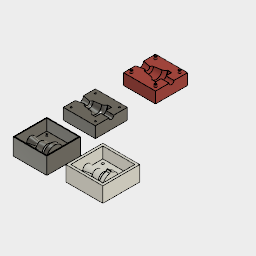
knobv8 (Autodesk Fusion 360 design; units mm, degrees)
Autodesk Fusion 360 part; units mm, degrees
sketch "Sketch1" plane through (0, 0, 0) normal (0, 0, 1) x (1, 0, 0)
  circle A0 centre (0, 0) radius 10
  line L0 (0, 13) -> (-1.5, 9.5)
  line L1 (-1.5, 9.5) -> (1.5, 9.5)
  line L2 (1.5, 9.5) -> (0, 13)
extrude "Extrude1" add sketch "Sketch1" along normal blind 5 makes body 1
sketch "Sketch2" plane through (0, 0, 5) normal (0, 0, 1) x (-1, 0, 0)
  arc A0 (1.3234, -9.912) -> (-1.3234, -9.912) centre (0, 0) ccw
  line L0 (-1.3234, -9.912) -> (0, -13)
  line L1 (0, -13) -> (1.3234, -9.912)
  circle A1 centre (0, 0) radius 7.5
  dimension "d3" = 15
  measures "d3" diameter of A1
ref_plane "WorkPlane1" through (0, 0, 20) normal (0, 0, 1) x (-1, 0, 0)
sketch "Sketch3" plane through (0, 0, 20) normal (0, 0, 1) x (1, 0, 0)
  circle A0 centre (0, 0) radius 5
loft "Loft1" add profiles "Sketch3", "Sketch2" section 1 section 2 contours A1 bodies 1
fillet "Fillet1" radius 0.5 3 edges at (0, -10, 5) (-0.6617, 11.456, 5) (0.6617, 11.456, 5) on bodies 1
fillet "Fillet2" radius 2.5 1 edges at (-4.6616, 1.8081, 20) on bodies 1
fillet "Fillet3" radius 5.5 1 edges at (6.9925, -2.7121, 5) on bodies 1
fillet "Fillet4" radius 0.5 2 edges at (0, 13, 2.25) (0, 12.6282, 4.8536) on bodies 1
sketch "Sketch5" plane through (0, 0, 0) normal (0, 0, -1) x (1, 0, 0)
  arc A0 (-0.4596, -11.9277) -> (0.4596, -11.9277) centre (0, -11.7307) ccw
  line L0 (0.4596, -11.9277) -> (1.3234, -9.912)
  arc A1 (1.3234, -9.912) -> (-1.3234, -9.912) centre (0, 0) ccw
  line L1 (-1.3234, -9.912) -> (-0.4596, -11.9277)
  line L2 (-15, 0) -> (15.3298, 0)
  line L3 (15.3298, 0) -> (15.3298, 10)
  line L4 (15.3298, 10) -> (-15, 10)
  line L5 (-15, 10) -> (-15, 0)
copy_body "CopyPasteBodies1" bodies 1 makes body 2
move_body "Move1" bodies 2 to x (1, 0, 0) y (0, 1, 0) z (0, 0, 1) at (-44, 0, 0)
extrude "Extrude3" cut sketch "Sketch5" along normal blind -22 and the other way blind -3 contours A1 L2 L4 L5 | A1 L2 | A1 L2 L3 L4 bodies 1
sketch "Sketch6" plane through (0, 0, 0) normal (0, 0, -1) x (1, 0, 0)
  arc A0 (-44.4596, -11.9277) -> (-43.5404, -11.9277) centre (-44, -11.7307) ccw
  line L0 (-43.5404, -11.9277) -> (-42.6766, -9.912)
  arc A1 (-42.6766, -9.912) -> (-45.3234, -9.912) centre (-44, 0) ccw
  line L1 (-45.3234, -9.912) -> (-44.4596, -11.9277)
  line L2 (-60, 0) -> (-30, 0)
  line L3 (-30, 0) -> (-30, -13)
  line L4 (-30, -13) -> (-60, -13)
  line L5 (-60, -13) -> (-60, 0)
extrude "Extrude4" cut sketch "Sketch6" along normal blind -22 and the other way blind -1 contours A0 L0 A1 L1 L2 | A0 L0 A1 L1 L2 L3 L4 L5 bodies 2
move_body "Move2" bodies 2 to x (1, 0, 0) y (0, 0, -1) z (0, 1, 0) at (0, -5, -5)
sketch "Sketch7" plane through (0, 0, 0) normal (0, 0, 1) x (1, 0, 0)
  line L0 (-65, 25) -> (-25, 25)
  line L1 (-25, 25) -> (-25, -15)
  line L2 (-25, -15) -> (-65, -15)
  line L3 (-65, -15) -> (-65, 25)
move_body "Align1" bodies 2 to x (0, 1, 0) y (-1, 0, 0) z (0, 0, 1) at (-70, 39, 5)
extrude "Extrude5" add sketch "Sketch7" against normal blind 5 separate body makes body 3
move_body "Align2" bodies 2 to x (1, 0, 0) y (0, 1, 0) z (0, 0, 1) at (30, 10, 0)
sketch "Sketch8" plane through (-65, 0, 0) normal (-1, 0, 0) x (0, -1, 0)
  line L0 (15, 0) -> (-25, 0)
  line L1 (-25, 0) -> (-25, -5)
  line L2 (-25, -5) -> (15, -5)
  line L3 (15, -5) -> (15, 0)
  circle A0 centre (-5, 0) radius 5
loft "Loft2" add profiles "Sketch8" section 1 contours L0 A0 picked at (-5.7088, 3.1054) section 2 face at (-55, 6.2273, 1.168) on bodies 2 bodies 2 3
move_body "Move3" bodies 1 to x (1, 0, 0) y (0, 1, 0) z (0, 0, 1) at (-43.1702, -52.4938, 0)
sketch "Sketch9" plane through (-35, 0, 0) normal (1, 0, 0) x (0, 1, 0)
  line L0 (-5, 0) -> (15, 0)
  arc A0 (15, 0) -> (-5, 0) centre (5, 0) ccw
  circle A1 centre (5, 0) radius 3
  dimension "d24" = 6
  measures "d24" diameter of A1
extrude "Extrude6" add sketch "Sketch9" along normal blind 10 contours L0 A1 picked at (5.9556, 0.2948) bodies 2
sketch "Sketch10" plane through (0, 0, -5) normal (0, 0, -1) x (1, 0, 0)
  line L0 (-25, 15) -> (-65, 15)
  line L1 (-65, 15) -> (-65, -25)
  line L2 (-65, -25) -> (-25, -25)
  line L3 (-25, -25) -> (-25, 15)
  line L4 (-75, 25) -> (-15, 25)
  line L5 (-15, 25) -> (-15, -35)
  line L6 (-15, -35) -> (-75, -35)
  line L7 (-75, -35) -> (-75, 25)
  line L8 (-78, -38) -> (-78, 28)
  line L9 (-78, 28) -> (-12, 28)
  line L10 (-12, 28) -> (-12, -38)
  line L11 (-12, -38) -> (-78, -38)
  dimension "d27" = 3
extrude "Extrude7" add sketch "Sketch10" against normal blind 15 contours L4 L5 L6 L7 bodies 2
sketch "Sketch11" plane through (0, 0, 0) normal (0, 0, 1) x (-1, 0, 0)
  line L0 (35, -8) -> (25, -8)
  line L1 (25, -8) -> (25, -25)
  line L2 (25, -25) -> (65, -25)
  line L3 (65, -25) -> (65, -10)
  line L4 (65, -10) -> (55, -7.8822)
  arc A0 (52.911, -10.3482) -> (55, -7.8822) centre (52.5, -7.8822) ccw
  line L5 (52.911, -10.3482) -> (43.9169, -11.8472)
  arc A1 (43.9169, -11.8472) -> (39.9434, -14.731) centre (44.8211, -17.2723) ccw
  arc A2 (39.5, -15) -> (39.9434, -14.731) centre (39.5, -14.5) ccw
  line L6 (39.5, -15) -> (35, -15)
  line L7 (35, -15) -> (35, -8)
  circle A3 centre (60, -20) radius 1
  circle A4 centre (30, -20) radius 1
  dimension "d39" = 2
  dimension "d40" = 2
  measures "d39" diameter of A4
  measures "d40" diameter of A3
sketch "Sketch12" plane through (0, 0, 0) normal (0, 0, 1) x (-1, 0, 0)
  line L0 (25, -2) -> (35, -2)
  line L1 (35, -2) -> (35, 5)
  line L2 (35, 5) -> (39.5, 5)
  arc A0 (39.9434, 4.731) -> (39.5, 5) centre (39.5, 4.5) ccw
  arc A1 (39.9434, 4.731) -> (43.9169, 1.8472) centre (44.8211, 7.2723) ccw
  line L3 (43.9169, 1.8472) -> (52.911, 0.3482)
  arc A2 (55, -2.1178) -> (52.911, 0.3482) centre (52.5, -2.1178) ccw
  line L4 (55, -2.1178) -> (65, 0)
  line L5 (65, 0) -> (65, 15)
  line L6 (65, 15) -> (25, 15)
  line L7 (25, 15) -> (25, -2)
  circle A3 centre (30, 10) radius 1
  circle A4 centre (60, 10) radius 1
  dimension "d37" = 2
  dimension "d38" = 2
  measures "d37" diameter of A3
  measures "d38" diameter of A4
extrude "Extrude8" add sketch "Sketch11" sketch "Sketch12" along normal blind 2 contours A3 | A4 of sketch 2 contours A3 | A4 bodies 2
fillet "Fillet5" radius 0.5 4 edges at (-59.0677, 20.3616, 2) (-59.0677, -9.6384, 2) (-29.0677, 20.3616, 2) (-29.0677, -9.6384, 2) on bodies 2
extrude "Extrude9" add 1 faces at (-71.6667, -1.6667, 10) along direction (0, 0, 1) blind 2 on bodies 2 bodies 2
sketch "Sketch13" plane through (0, 0, 12) normal (0, 0, 1) x (-1, 0, 0)
  line L0 (25, -25) -> (25, 15)
  line L1 (25, 15) -> (65, 15)
  line L2 (65, 15) -> (65, -25)
  line L3 (65, -25) -> (25, -25)
  line L4 (15, -35) -> (75, -35)
  line L5 (75, -35) -> (75, 25)
  line L6 (75, 25) -> (15, 25)
  line L7 (15, 25) -> (15, -35)
  line L8 (65, -25) -> (25, -25)
  line L9 (25, -25) -> (25, 15)
  line L10 (25, 15) -> (65, 15)
  line L11 (65, 15) -> (65, -25)
extrude "Extrude10" add sketch "Sketch13" against normal blind 12 separate body contours L0 L1 L2 L3 L8 L9 L10 L11 makes body 4
combine "Combine1" operation cut target body 4 tool bodies 2 keep tools
move_body "Move4" bodies 4 to x (1, 0, 0) y (0, -1, 0) z (0, 0, -1) at (-6.4144, 76.1132, 21)
move_body "Align3" bodies 2 to x (1, 0, 0) y (0, 1, 0) z (0, 0, 1) at (0, 16.1132, 14)
move_body "Move5" bodies 2 to x (1, 0, 0) y (0, 1, 0) z (0, 0, 1) at (0, -6, 0)
move_body "Move6" bodies 1 to x (0, -1, 0) y (0, 0, 1) z (-1, 0, 0) at (-53.1702, -105.664, 52.4938)
move_body "Align4" bodies 1 to x (1, 0, 0) y (0, 1, 0) z (0, 0, 1) at (0, 0, 14)
move_body "Align5" bodies 1 to x (1, 0, 0) y (0, 1, 0) z (0, 0, 1) at (18.1702, 0, 0)
sketch "Sketch14" plane through (0, 0, 0) normal (0, 0, 1) x (1, 0, 0)
  line L0 (-70, -85) -> (-30, -85)
  line L1 (-30, -85) -> (-30, -45)
  line L2 (-30, -45) -> (-70, -45)
  line L3 (-70, -45) -> (-70, -85)
  dimension "d41" = 40
  dimension "d42" = 40
  measures "d41" distance of L0.start L0.end
  measures "d42" distance of L0.start L2.end
extrude "Extrude11" add sketch "Sketch14" along normal blind 3 separate body makes body 5
move_body "Align6" bodies 5 to x (1, 0, 0) y (0, 1, 0) z (0, 0, 1) at (5, 2.5062, 14)
move_body "Move7" bodies 5 to x (1, 0, 0) y (0, 1, 0) z (0, 0, 1) at (0, 0, -3)
sketch "Sketch15" plane through (-35, 0, 0) normal (1, 0, 0) x (0, 1, 0)
  line L0 (-72.4938, 14) -> (-52.4938, 14)
  arc A0 (-52.4938, 14) -> (-61.1704, 23.912) centre (-62.4938, 14) ccw
  line L1 (-61.1704, 23.912) -> (-62.0343, 25.9277)
  arc A1 (-62.0343, 25.9277) -> (-62.9534, 25.9277) centre (-62.4938, 25.7307) ccw
  line L2 (-62.9534, 25.9277) -> (-63.8172, 23.912)
  arc A2 (-63.8172, 23.912) -> (-72.4938, 14) centre (-62.4938, 14) ccw
  circle A3 centre (-62.4938, 14) radius 3
  dimension "d45" = 6
  measures "d45" diameter of A3
extrude "Extrude12" add sketch "Sketch15" along normal blind 10 contours L0 A3 picked at (-63.3259, 15.1141) bodies 1 5
sketch "Sketch16" plane through (-55, 0, 0) normal (-1, 0, 0) x (0, -1, 0)
  line L0 (59.6116, 14) -> (65.376, 14)
  arc A0 (65.376, 14) -> (59.6116, 14) centre (62.4938, 14) ccw
sketch "Sketch17" plane through (-65, 0, 0) normal (-1, 0, 0) x (0, -1, 0)
  line L0 (42.4938, 11) -> (82.4938, 11)
  line L1 (82.4938, 11) -> (82.4938, 14)
  line L2 (82.4938, 14) -> (42.4938, 14)
  line L3 (42.4938, 14) -> (42.4938, 11)
  circle A0 centre (62.4938, 14) radius 5
  point P0 (62.4938, 14)
  dimension "d48" = 10
  measures "d48" diameter of A0
loft "Loft3" add profiles "Sketch17", "Sketch16" section 1 contours L2 A0 section 2 bodies 1
extrude "Extrude13" add 1 faces at (-71.6667, 8.4465, 26) along direction (0, 0, 1) blind 2 on bodies 2 bodies 2
move_body "Move8" bodies 1 to x (1, 0, 0) y (0, 1, 0) z (0, 0, 1) at (-0.5044, 1.7197, 0)
move_body "Move9" bodies 1 to x (1, 0, 0) y (0, 1, 0) z (0, 0, 1) at (65.5044, 80.7741, 0)
sketch "Sketch18" plane through (0, 0, 14) normal (0, 0, 1) x (-1, 0, 0)
  line L0 (-10, -17.1178) -> (0, -15)
  line L1 (0, -15) -> (0, 0)
  line L2 (0, 0) -> (-40, 0)
  line L3 (-40, 0) -> (-40, -17)
  line L4 (-40, -17) -> (-30, -17)
  line L5 (-30, -17) -> (-30, -10)
  line L6 (-30, -10) -> (-25.5, -10)
  arc A0 (-25.0566, -10.269) -> (-25.5, -10) centre (-25.5, -10.5) ccw
  arc A1 (-25.0566, -10.269) -> (-21.0831, -13.1528) centre (-20.1789, -7.7277) ccw
  line L7 (-21.0831, -13.1528) -> (-12.089, -14.6518)
  arc A2 (-10, -17.1178) -> (-12.089, -14.6518) centre (-12.5, -17.1178) ccw
  circle A3 centre (-35, -5) radius 1.5
  circle A4 centre (-5, -5) radius 1.5
  circle A5 centre (-5, -35) radius 1.5
  circle A6 centre (-35, -35) radius 1.5
  dimension "d54" = 3
  dimension "d55" = 3
  dimension "d56" = 3
  dimension "d57" = 3
  measures "d54" diameter of A3
  measures "d55" diameter of A4
  measures "d56" diameter of A5
  measures "d57" diameter of A6
extrude "Extrude14" add 1 faces at (13.3333, 26.6667, 11) along direction (0, 0, -1) blind 1 on bodies 1 bodies 1
extrude "Extrude15" add 1 faces at (13.3333, 26.6667, 10) along direction (0, 0, -1) blind 1 on bodies 1 bodies 1
extrude "Extrude16" cut sketch "Sketch18" against normal blind 3 contours A3 | A4 | A5 | A6 bodies 1
fillet "Fillet6" radius 0.5 4 edges at (36.3985, 4.4576, 11) (36.3985, 34.4576, 11) (6.3985, 34.4576, 11) (6.3985, 4.4576, 11) on bodies 1
sketch "Sketch19" plane through (0, 0, 14) normal (0, 0, 1) x (-1, 0, 0)
  circle A0 centre (-5, -5) radius 1.5
  circle A1 centre (-35, -5) radius 1.5
  line L0 (-10, -17.1178) -> (0, -15)
  line L1 (0, -15) -> (0, 0)
  line L2 (0, 0) -> (-40, 0)
  line L3 (-40, 0) -> (-40, -17)
  line L4 (-40, -17) -> (-30, -17)
  line L5 (-30, -17) -> (-30, -10)
  line L6 (-30, -10) -> (-25.5, -10)
  arc A2 (-25.0566, -10.269) -> (-25.5, -10) centre (-25.5, -10.5) ccw
  arc A3 (-25.0566, -10.269) -> (-21.0831, -13.1528) centre (-20.1789, -7.7277) ccw
  line L7 (-21.0831, -13.1528) -> (-12.089, -14.6518)
  arc A4 (-10, -17.1178) -> (-12.089, -14.6518) centre (-12.5, -17.1178) ccw
  line L8 (0, -40) -> (-40, -40)
  line L9 (-40, -40) -> (-40, 0)
  line L10 (-40, 0) -> (0, 0)
  line L11 (0, 0) -> (0, -40)
  line L12 (-43, 3) -> (3, 3)
  line L13 (3, 3) -> (3, -43)
  line L14 (3, -43) -> (-43, -43)
  line L15 (-43, -43) -> (-43, 3)
  point P0 (0, -40)
  dimension "d65" = 3
extrude "Extrude17" add sketch "Sketch19" along normal blind 14 and the other way blind 5 contours L12 L13 L14 L15 bodies 1
sketch "Sketch20" plane through (0, 0, 28) normal (0, 0, 1) x (-1, 0, 0)
  line L0 (-40, 0) -> (0, 0)
  line L1 (0, 0) -> (0, -40)
  line L2 (0, -40) -> (-40, -40)
  line L3 (-40, -40) -> (-40, 0)
  line L4 (-43, -43) -> (3, -43)
  line L5 (3, -43) -> (3, 3)
  line L6 (3, 3) -> (-43, 3)
  line L7 (-43, 3) -> (-43, -43)
  line L8 (0, -40) -> (-40, -40)
  line L9 (-40, -40) -> (-40, 0)
  line L10 (-40, 0) -> (0, 0)
  line L11 (0, 0) -> (0, -40)
extrude "Extrude18" add sketch "Sketch20" against normal blind 17 separate body contours L0 L1 L2 L3 L8 L9 L10 L11 makes body 6
combine "Combine2" operation cut target body 6 tool bodies 1 keep tools
move_body "Move10" bodies 6 to x (1, 0, 0) y (0, -1, 0) z (0, 0, -1) at (-36.3709, 87.8255, 22)
move_body "Align7" bodies 6 to x (1, 0, 0) y (0, 1, 0) z (0, 0, 1) at (-35.0435, 43.2877, 15)
move_body "Move11" bodies 6 to x (1, 0, 0) y (0, 1, 0) z (0, 0, 1) at (0, 7, 0)
extrude "Extrude19" add 1 faces at (-44.7477, 77.7798, 9) along direction (0, 0, -1) blind 2 on bodies 4 bodies 4
move_body "Align8" bodies 4 to x (1, 0, 0) y (0, 1, 0) z (0, 0, 1) at (0, 7, 2)
move_body "Move12" bodies 6 to x (1, 0, 0) y (0, 1, 0) z (0, 0, 1) at (0, 4, 0)
move_body "Move13" bodies 4 to x (1, 0, 0) y (0, -1, 0) z (0, 0, -1) at (-12.4211, 152.2641, 18)
move_body "Align9" bodies 4 to x (1, 0, 0) y (0, 1, 0) z (0, 0, 1) at (12.4211, 0, 28)
move_body "Align10" bodies 4 to x (1, 0, 0) y (0, 1, 0) z (0, 0, 1) at (0, 47.9622, 0)
sketch "Sketch21" plane through (-25, 0, 0) normal (-1, 0, 0) x (0, -1, 0)
  line L0 (-35.1132, 14) -> (-18.1132, 14)
  arc A0 (-12.1132, 14) -> (-18.1132, 14) centre (-15.1132, 14) ccw
  line L1 (-12.1132, 14) -> (4.8868, 14)
  line L2 (4.8868, 14) -> (4.8868, 28)
  line L3 (4.8868, 28) -> (-35.1132, 28)
  line L4 (-35.1132, 28) -> (-35.1132, 14)
  line L5 (-12.1132, 15.7321) -> (-15.1132, 17.4641)
  line L6 (-15.1132, 17.4641) -> (-18.1132, 15.7321)
  line L7 (-18.1132, 15.7321) -> (-18.1132, 12.2679)
  line L8 (-18.1132, 12.2679) -> (-15.1132, 10.5359)
  line L9 (-15.1132, 10.5359) -> (-12.1132, 12.2679)
  line L10 (-12.1132, 12.2679) -> (-12.1132, 15.7321)
  line L11 (-10.1132, 16.8868) -> (-15.1132, 19.7735)
  line L12 (-15.1132, 19.7735) -> (-20.1132, 16.8868)
  line L13 (-20.1132, 16.8868) -> (-20.1132, 11.1132)
  line L14 (-20.1132, 11.1132) -> (-15.1132, 8.2265)
  line L15 (-15.1132, 8.2265) -> (-10.1132, 11.1132)
  line L16 (-10.1132, 11.1132) -> (-10.1132, 16.8868)
  point P0 (-15.1132, 14)
  dimension "d74" = 2
extrude "Extrude20" add 1 faces at (-55, 5.1132, 9) along direction (0, 0, -1) blind 2 on bodies 2 bodies 2
extrude "Extrude21" add sketch "Sketch21" along normal blind 6.5 and the other way blind -1.5 contours L0 L1 L5 L6 L7 L10 L11 L12 L13 L16 | A0 L6 L7 | A0 L5 L6 | A0 L5 L10 bodies 2
sketch "Sketch22" plane through (0, 0, 28) normal (0, 0, 1) x (-1, 0, 0)
  line L0 (25, -35.1132) -> (25, 4.8868)
  line L1 (25, 4.8868) -> (65, 4.8868)
  line L2 (65, 4.8868) -> (65, -35.1132)
  line L3 (65, -35.1132) -> (25, -35.1132)
  line L4 (15, -45.1132) -> (75, -45.1132)
  line L5 (75, -45.1132) -> (75, 14.8868)
  line L6 (75, 14.8868) -> (15, 14.8868)
  line L7 (15, 14.8868) -> (15, -45.1132)
  line L8 (65, -35.1132) -> (25, -35.1132)
  line L9 (25, -35.1132) -> (25, 4.8868)
  line L10 (25, 4.8868) -> (65, 4.8868)
  line L11 (65, 4.8868) -> (65, -35.1132)
extrude "Extrude22" add sketch "Sketch22" against normal blind 14 separate body contours L0 L1 L2 L3 L8 L9 L10 L11 makes body 7
combine "Combine3" operation cut target body 7 tool bodies 2 keep tools
move_body "Move14" bodies 7 to x (-1, 0, 0) y (0, 1, 0) z (0, 0, -1) at (-130, 0, 80)
sketch "Sketch23" plane through (40, 0, 0) normal (-1, 0, 0) x (0, -1, 0)
  line L0 (-17, 14) -> (0, 14)
  line L1 (0, 14) -> (0, 28)
  line L2 (0, 28) -> (-40, 28)
  line L3 (-40, 28) -> (-40, 14)
  line L4 (-40, 14) -> (-23, 14)
  arc A0 (-17, 14) -> (-23, 14) centre (-20, 14) ccw
  line L5 (-17, 15.7321) -> (-20, 17.4641)
  line L6 (-20, 17.4641) -> (-23, 15.7321)
  line L7 (-23, 15.7321) -> (-23, 12.2679)
  line L8 (-23, 12.2679) -> (-20, 10.5359)
  line L9 (-20, 10.5359) -> (-17, 12.2679)
  line L10 (-17, 12.2679) -> (-17, 15.7321)
  line L11 (-25, 16.8868) -> (-25, 11.1132)
  line L12 (-25, 11.1132) -> (-20, 8.2265)
  line L13 (-20, 8.2265) -> (-15, 11.1132)
  line L14 (-15, 11.1132) -> (-15, 16.8868)
  line L15 (-15, 16.8868) -> (-20, 19.7735)
  line L16 (-20, 19.7735) -> (-25, 16.8868)
  point P0 (-20, 14)
  dimension "d83" = 2
extrude "Extrude23" add sketch "Sketch23" along normal blind 6.5 and the other way blind -1.5 contours L0 L4 L5 L6 L7 L10 L11 L14 L15 L16 | A0 L5 L10 | A0 L5 L6 | A0 L6 L7 bodies 1
sketch "Sketch24" plane through (0, 0, 28) normal (0, 0, 1) x (-1, 0, 0)
  line L0 (-40, 0) -> (0, 0)
  line L1 (0, 0) -> (0, -40)
  line L2 (0, -40) -> (-40, -40)
  line L3 (-40, -40) -> (-40, 0)
  line L4 (-43, -43) -> (3, -43)
  line L5 (3, -43) -> (3, 3)
  line L6 (3, 3) -> (-43, 3)
  line L7 (-43, 3) -> (-43, -43)
  line L8 (0, -40) -> (-40, -40)
  line L9 (-40, -40) -> (-40, 0)
  line L10 (-40, 0) -> (0, 0)
  line L11 (0, 0) -> (0, -40)
extrude "Extrude24" add sketch "Sketch24" against normal blind 14 separate body contours L0 L1 L2 L3 L8 L9 L10 L11 makes body 8
combine "Combine4" operation cut target body 8 tool bodies 1 keep tools
move_body "Move15" bodies 8 to x (-1, 0, 0) y (0, 1, 0) z (0, 0, -1) at (0, 0, 77)
sketch "Sketch25" plane through (0, 0, 0) normal (0, 0, 1) x (1, 0, 0)
  line L0 (0, -25) -> (88, -25)
  line L1 (88, -25) -> (88, -205)
  line L2 (88, -205) -> (0, -205)
  line L3 (0, -205) -> (0, -25)
  dimension "d90" = 88
  dimension "d91" = 180
  measures "d90" distance of L0.start L0.end
  measures "d91" distance of L0.start L2.end
extrude "Extrude26" cut 1 faces at (-55, -14.8868, 14) along direction (0, 1, 0) blind 9 on bodies 2 bodies 2
extrude "Extrude27" cut 1 faces at (-15, 11.1132, 21) along direction (-1, 0, 0) blind 9 on bodies 2 bodies 2
extrude "Extrude28" cut 1 faces at (-41, 45.1132, 21) along direction (0, -1, 0) blind 9 on bodies 2 bodies 2
extrude "Extrude29" cut 1 faces at (-75, 22.1132, 14) along direction (1, 0, 0) blind 9 on bodies 2 bodies 2
move_body "Move16" bodies 4 to x (1, 0, 0) y (0, -1, 0) z (0, 0, -1) at (0, 204.2263, 46)
move_body "Move17" bodies 6 to x (1, 0, 0) y (0, 1, 0) z (0, 0, 1) at (0, 35, 0)
hidden bodies 7 8
equation "diametre = 6 mm"
equation "d24 = diametre"
equation "d45 = diametre"
equation "d70 = -14 mm - 3 mm"
